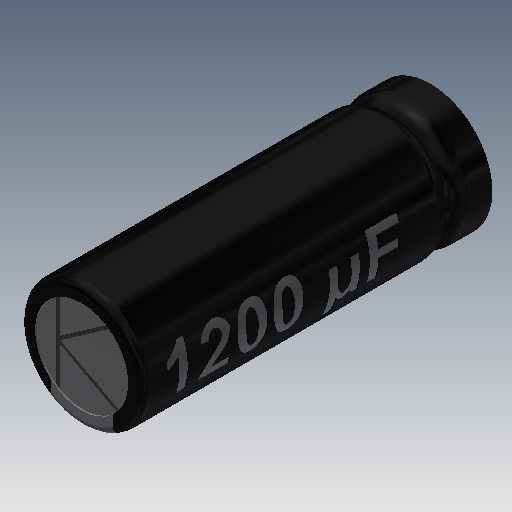
# Autodesk Inventor part: config - capasitor 1200 μF
Saved by Autodesk Inventor 2020 (Build 240152000, 152)
## iProperties
Created: 2005-12-06
Part Number: config - capasitor 1200 μF
Document SubType Name: Modeling
Designer: Simon.Ng@autodesk.com
Stock Number: config - capasitor 1200 μF
Density: 1 g/cm^3
Material: Generic
Mass: 1.11838 g
Surface Area: 6.73435 cm^2
Volume: 1.11838 cm^3
Appearance: Glossy - Black
Company: Autodesk Asia Pte. Ltd.
Title: PC Demo
Author: Simon.Ng@autodesk.com
Autodesk Inventor part; units mm, degrees
ref_plane "YZ Plane" through (0, 0, 0) normal (1, 0, 0) x (0, 1, 0)
ref_plane "XZ Plane" through (0, 0, 0) normal (0, 1, 0) x (-1, 0, 0)
sketch "Sketch1" plane through (0, 0, 0) normal (0, 0, 1) x (1, 0, 0)
  line L0 (0, 6.4) -> (0, -4.8) construction
  line L1 (-4.8, 0) -> (6.4, 0) construction
  circle A0 centre (0, 0) radius 4
  dimension "d0" = 8
  constraints: 2 point on line, 1 centre point
  measures "d0" diameter of A0
extrude "Extrusion1" add sketch "Sketch1" along normal blind 22.5
sketch "Sketch6" plane through (0, 0, 0) normal (1, 0, 0) x (0, 1, 0)
  line L0 (0, 29.25) -> (0, -2.25) projected
  line L1 (4, 0) -> (4, 22.5) projected
  line L2 (4, 3.5) -> (4, 1.5)
  line L3 (4, 2.5) -> (3.5, 2.5) construction
  line L4 (-4, 0) -> (4, 0) construction
  arc A0 (3.5, 2.5) -> (4, 3.5) centre (2.75, 3.5) ccw
  arc A1 (4, 1.5) -> (3.5, 2.5) centre (2.75, 1.5) ccw
  point P0 (0, 0)
  dimension "d16" = 2
  dimension "d17" = 2.5
  dimension "d18" = 0.5
  constraints: 4 end point, 4 point on circle, 2 centre point, 2 point on line, 2 tangent, 1 collinear, 1 horizontal, 1 midpoint
  measures "d16" distance of L2.start L2.end
  measures "d17" distance between parallel lines of L4 L3
  measures "d18" distance of L3.start L3.end
revolve "Revolution1" cut sketch "Sketch6" angle 360 about axis through (0, 0, 0) along (0, 0, -1)
sketch "Sketch2" plane through (0, 0, 22.5) normal (0, 0, 1) x (1, 0, 0)
  circle A0 centre (0, 0) radius 4 projected
  circle A1 centre (0, 0) radius 3
  dimension "d3" = 1
  constraints: 1 centre point, 1 coincident
  measures "d3" radial gap between concentric circles of A1 A0
extrude "Extrusion2" cut sketch "Sketch2" against normal blind 0.1 contours A1
sketch "Sketch3" plane through (0, 0, 22.4) normal (0, 0, 1) x (1, 0, 0)
  line L0 (-1.7345, 2.8958) -> (-1.4712, 2.8958)
  line L1 (-1.4712, 2.8958) -> (-1.4712, -3.0531)
  line L2 (-1.4712, -3.0531) -> (-1.7345, -3.0531)
  line L3 (-1.7345, -3.0531) -> (-1.7345, 2.8958)
  line L4 (-1.4712, 0.1227) -> (-1.5962, 0.3017)
  line L5 (-1.5962, 0.3017) -> (1.7965, 2.6719)
  line L6 (1.7965, 2.6719) -> (1.9215, 2.493)
  line L7 (1.9215, 2.493) -> (-1.4712, 0.1227)
  line L8 (-1.4712, 0.1227) -> (-1.5776, -0.0787)
  line L9 (-1.5776, -0.0787) -> (2.3639, -2.1618)
  line L10 (2.3639, -2.1618) -> (2.4704, -1.9604)
  line L11 (2.4704, -1.9604) -> (-1.4712, 0.1227)
  constraints: 24 end point, 6 parallel, 3 perpendicular, 1 horizontal, 1 point on line
extrude "Extrusion3" cut sketch "Sketch3" against normal blind 0.05
fillet "Fillet1" radius 0.5 1 edges at (-4, 0, 22.5)
sketch "Sketch5" plane through (0, 0, 22.5) normal (0, 0, 1) x (1, 0, 0)
  circle A0 centre (0, 0) radius 3 projected
  circle A1 centre (0, 0) radius 4 projected
  line L0 (2, -2.2361) -> (2, -5)
  line L1 (2, -5) -> (-2, -5)
  line L2 (-2, -5) -> (-2, -2.2361)
  line L3 (0, -4.8) -> (0, 6.4) projected
  point P0 (0, -4)
  point P1 (0, -4)
  dimension "d12" = 1
  dimension "d13" = 4
  constraints: 6 end point, 2 point on circle, 1 coincident, 1 parallel, 1 point on line, 1 vertical alignment, 2 other
  measures "d12" distance from line of L1 point (0, -4)
  measures "d13" distance of L0.end L1.end
split_face "Split1"
ref_plane "Work Plane1" through (10, 0, 0) normal (1, 0, 0) x (0, 1, 0)
sketch "Sketch4" plane through (10, 0, 0) normal (1, 0, 0) x (0, 0, -1)
  line L0 (-21.2563, 1.6353) -> (-5.6481, 1.6353) construction
  line L1 (-5.6481, 1.6353) -> (-5.6481, -2.2039) construction
  line L2 (-5.6481, -2.2039) -> (-21.2563, -2.2039) construction
  line L3 (-21.2563, -2.2039) -> (-21.2563, 1.6353) construction
  line L4 (-19.6054, -1.3762) -> (-20.1816, -1.3762)
  line L5 (-20.1816, -1.3762) -> (-20.1816, 0.7892)
  spline S0 degree 2 poles (-20.1816, 0.7892) (-20.4972, 0.4966) (-20.9248, 0.3548) knots 0 0 0 1 1 1
  line L6 (-20.9248, 0.3548) -> (-20.9248, 0.8761)
  spline S1 degree 3 poles (-20.9248, 0.8761) (-20.6984, 0.9493) (-20.1702, 1.3609) (-20.0719, 1.6353) knots 0 0 0 0 1 1 1 1
  line L7 (-20.0719, 1.6353) -> (-19.6054, 1.6353)
  line L8 (-19.6054, 1.6353) -> (-19.6054, -1.3762)
  line L9 (-16.8066, -0.8411) -> (-16.8066, -1.3762)
  line L10 (-16.8066, -1.3762) -> (-18.8211, -1.3762)
  spline S2 degree 3 poles (-18.8211, -1.3762) (-18.7891, -1.0743) (-18.4621, -0.5324) (-17.9774, -0.0842) knots 0 0 0 0 1 1 1 1
  spline S3 degree 2 poles (-17.9774, -0.0842) (-17.5886, 0.277) (-17.5018, 0.4074) knots 0 0 0 1 1 1
  spline S4 degree 2 poles (-17.5018, 0.4074) (-17.3829, 0.5857) (-17.3829, 0.7595) knots 0 0 0 1 1 1
  spline S5 degree 3 poles (-17.3829, 0.7595) (-17.3829, 0.9516) (-17.5886, 1.1574) (-17.7716, 1.1574) knots 0 0 0 0 1 1 1 1
  spline S6 degree 3 poles (-17.7716, 1.1574) (-17.9499, 1.1574) (-18.1626, 0.9402) (-18.1786, 0.6886) knots 0 0 0 0 1 1 1 1
  line L11 (-18.1786, 0.6886) -> (-18.7525, 0.7458)
  spline S7 degree 3 poles (-18.7525, 0.7458) (-18.7022, 1.2214) (-18.1626, 1.6353) (-17.7579, 1.6353) knots 0 0 0 0 1 1 1 1
  spline S8 degree 3 poles (-17.7579, 1.6353) (-17.3143, 1.6353) (-16.8066, 1.1574) (-16.8066, 0.8007) knots 0 0 0 0 1 1 1 1
  spline S9 degree 3 poles (-16.8066, 0.8007) (-16.8066, 0.5995) (-16.9507, 0.2336) (-17.1085, 0.0324) knots 0 0 0 0 1 1 1 1
  spline S10 degree 4 poles (-17.1085, 0.0324) (-17.2136, -0.1002) (-17.7579, -0.5987) (-17.9042, -0.7633) (-17.9476, -0.8411) knots 0 0 0 0 0 1 1 1 1 1
  line L12 (-17.9476, -0.8411) -> (-16.8066, -0.8411)
  spline S11 degree 2 poles (-15.4461, 1.6353) (-15.0094, 1.6353) (-14.7647, 1.3243) knots 0 0 0 1 1 1
  spline S12 degree 2 poles (-14.7647, 1.3243) (-14.472, 0.9562) (-14.472, 0.1033) knots 0 0 0 1 1 1
  spline S13 degree 2 poles (-14.472, 0.1033) (-14.472, -0.7473) (-14.767, -1.1201) knots 0 0 0 1 1 1
  spline S14 degree 2 poles (-14.767, -1.1201) (-15.0094, -1.4265) (-15.4461, -1.4265) knots 0 0 0 1 1 1
  spline S15 degree 3 poles (-15.4461, -1.4265) (-15.8851, -1.4265) (-16.4202, -0.7542) (-16.4202, 0.1101) knots 0 0 0 0 1 1 1 1
  spline S16 degree 2 poles (-16.4202, 0.1101) (-16.4202, 0.9562) (-16.1252, 1.3289) knots 0 0 0 1 1 1
  spline S17 degree 2 poles (-16.1252, 1.3289) (-15.8829, 1.6353) (-15.4461, 1.6353) knots 0 0 0 1 1 1
  spline S18 degree 3 poles (-15.4461, 1.1574) (-15.5513, 1.1574) (-15.7136, 1.0248) (-15.7594, 0.8533) knots 0 0 0 0 1 1 1 1
  spline S19 degree 2 poles (-15.7594, 0.8533) (-15.8188, 0.6315) (-15.8188, 0.1033) knots 0 0 0 1 1 1
  spline S20 degree 4 poles (-15.8188, 0.1033) (-15.8188, -0.4226) (-15.7114, -0.8182) (-15.5513, -0.9486) (-15.4461, -0.9486) knots 0 0 0 0 0 1 1 1 1 1
  spline S21 degree 3 poles (-15.4461, -0.9486) (-15.3409, -0.9486) (-15.1786, -0.8159) (-15.1329, -0.6444) knots 0 0 0 0 1 1 1 1
  spline S22 degree 2 poles (-15.1329, -0.6444) (-15.0734, -0.4226) (-15.0734, 0.1033) knots 0 0 0 1 1 1
  spline S23 degree 4 poles (-15.0734, 0.1033) (-15.0734, 0.6315) (-15.1809, 1.0248) (-15.3409, 1.1574) (-15.4461, 1.1574) knots 0 0 0 0 0 1 1 1 1 1
  spline S24 degree 2 poles (-13.1161, 1.6353) (-12.6794, 1.6353) (-12.4347, 1.3243) knots 0 0 0 1 1 1
  spline S25 degree 2 poles (-12.4347, 1.3243) (-12.142, 0.9562) (-12.142, 0.1033) knots 0 0 0 1 1 1
  spline S26 degree 2 poles (-12.142, 0.1033) (-12.142, -0.7473) (-12.437, -1.1201) knots 0 0 0 1 1 1
  spline S27 degree 2 poles (-12.437, -1.1201) (-12.6794, -1.4265) (-13.1161, -1.4265) knots 0 0 0 1 1 1
  spline S28 degree 3 poles (-13.1161, -1.4265) (-13.5551, -1.4265) (-14.0902, -0.7542) (-14.0902, 0.1101) knots 0 0 0 0 1 1 1 1
  spline S29 degree 2 poles (-14.0902, 0.1101) (-14.0902, 0.9562) (-13.7952, 1.3289) knots 0 0 0 1 1 1
  spline S30 degree 2 poles (-13.7952, 1.3289) (-13.5528, 1.6353) (-13.1161, 1.6353) knots 0 0 0 1 1 1
  spline S31 degree 3 poles (-13.1161, 1.1574) (-13.2213, 1.1574) (-13.3836, 1.0248) (-13.4294, 0.8533) knots 0 0 0 0 1 1 1 1
  spline S32 degree 2 poles (-13.4294, 0.8533) (-13.4888, 0.6315) (-13.4888, 0.1033) knots 0 0 0 1 1 1
  spline S33 degree 4 poles (-13.4888, 0.1033) (-13.4888, -0.4226) (-13.3813, -0.8182) (-13.2213, -0.9486) (-13.1161, -0.9486) knots 0 0 0 0 0 1 1 1 1 1
  spline S34 degree 3 poles (-13.1161, -0.9486) (-13.0109, -0.9486) (-12.8486, -0.8159) (-12.8028, -0.6444) knots 0 0 0 0 1 1 1 1
  spline S35 degree 2 poles (-12.8028, -0.6444) (-12.7434, -0.4226) (-12.7434, 0.1033) knots 0 0 0 1 1 1
  spline S36 degree 4 poles (-12.7434, 0.1033) (-12.7434, 0.6315) (-12.8508, 1.0248) (-13.0109, 1.1574) (-13.1161, 1.1574) knots 0 0 0 0 0 1 1 1 1 1
  line L13 (-10.4774, 0.7984) -> (-9.9011, 0.7984)
  line L14 (-9.9011, 0.7984) -> (-9.9011, -0.1894)
  spline S37 degree 4 poles (-9.9011, -0.1894) (-9.9011, -0.4661) (-9.844, -0.7771) (-9.6428, -0.9691) (-9.501, -0.9691) knots 0 0 0 0 0 1 1 1 1 1
  spline S38 degree 4 poles (-9.501, -0.9691) (-9.3547, -0.9691) (-9.142, -0.7679) (-9.0803, -0.4821) (-9.0803, -0.1963) knots 0 0 0 0 0 1 1 1 1 1
  line L15 (-9.0803, -0.1963) -> (-9.0803, 0.7984)
  line L16 (-9.0803, 0.7984) -> (-8.504, 0.7984)
  line L17 (-8.504, 0.7984) -> (-8.504, -1.3762)
  line L18 (-8.504, -1.3762) -> (-9.0345, -1.3762)
  line L19 (-9.0345, -1.3762) -> (-9.0345, -1.1132)
  spline S39 degree 2 poles (-9.0345, -1.1132) (-9.1946, -1.4242) (-9.4713, -1.4242) knots 0 0 0 1 1 1
  spline S40 degree 2 poles (-9.4713, -1.4242) (-9.764, -1.4242) (-9.9011, -1.1132) knots 0 0 0 1 1 1
  line L20 (-9.9011, -1.1132) -> (-9.9011, -2.2039)
  line L21 (-9.9011, -2.2039) -> (-10.4774, -2.2039)
  line L22 (-10.4774, -2.2039) -> (-10.4774, 0.7984)
  line L23 (-7.9027, -1.3762) -> (-7.9027, 1.6238)
  line L24 (-7.9027, 1.6238) -> (-5.8425, 1.6238)
  line L25 (-5.8425, 1.6238) -> (-5.8425, 1.1162)
  line L26 (-5.8425, 1.1162) -> (-7.2967, 1.1162)
  line L27 (-7.2967, 1.1162) -> (-7.2967, 0.4074)
  line L28 (-7.2967, 0.4074) -> (-6.0414, 0.4074)
  line L29 (-6.0414, 0.4074) -> (-6.0414, -0.1002)
  line L30 (-6.0414, -0.1002) -> (-7.2967, -0.1002)
  line L31 (-7.2967, -0.1002) -> (-7.2967, -1.3762)
  line L32 (-7.2967, -1.3762) -> (-7.9027, -1.3762)
  constraints: 2 other
emboss "Emboss1" sketch "Sketch4" operation cut depth 0.05 direction (1, 0, 0) wrap yes faces at (-0.4906, 3.9698, 9.6667) (3.9468, -0.6414, 22.0374) (-0.4906, 3.9698, 1)
body "Solid1"
